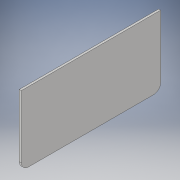
# Autodesk Inventor part: Part1
Saved by Autodesk Inventor 2019 (Build 230136000, 136)
## iProperties
Created: 2019-08-08
Part Number: Part1
Material: Generic
Document SubType Name: Modeling
Designer: daozhou.cen
Density: 1 g/cm^3
Appearance: Default
Author: daozhou.cen
Autodesk Inventor part; units mm, degrees
ref_plane "YZ Plane" through (0, 0, 0) normal (1, 0, 0) x (0, 1, 0)
ref_plane "XZ Plane" through (0, 0, 0) normal (0, 1, 0) x (-1, 0, 0)
ref_plane "XY Plane" through (0, 0, 0) normal (0, 0, 1) x (1, 0, 0)
sketch "Sketch1" plane through (0, 0, 0) normal (1, 0, 0) x (0, 1, 0)
  line L0 (-50, 100) -> (50, 100) construction
  line L1 (50, 100) -> (50, -100) construction
  line L2 (50, -100) -> (-50, -100) construction
  line L3 (-50, -100) -> (-50, 100) construction
  line L4 (-50, 100) -> (50, -100) construction
  line L5 (50, 100) -> (-50, -100) construction
  line L6 (50, 100) -> (-40, 100)
  line L7 (50, -100) -> (-40, -100)
  arc A0 (-40, 100) -> (-50, 90) centre (-40, 90) ccw
  arc A1 (-50, -90) -> (-40, -100) centre (-40, -90) ccw
  line L8 (-50, -90) -> (-50, 90)
  line L9 (50, 100) -> (50, -100)
  point P0 (0, 0)
  dimension "d0" = 100
  dimension "d1" = 200
  dimension "d2" = 90
  dimension "d3" = 90
  constraints: 20 end point, 4 point on circle, 4 point on line, 4 tangent, 2 centre point, 2 midpoint, 2 parallel, 2 perpendicular, 1 collinear, 1 horizontal
  measures "d0" distance of L1.end L2.end
  measures "d1" distance of L0.end L1.end
  measures "d2" distance of L0.end L6.end
  measures "d3" distance of L1.end L7.end
extrude "Extrusion1" add sketch "Sketch1" along normal blind 3
equation "\"d3\" = d2"
body "Solid1"
